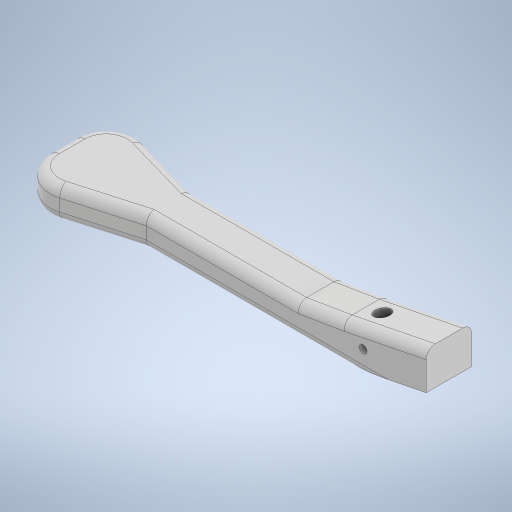
# Autodesk Inventor part: ручка печать
Saved by Autodesk Inventor 2023 (Build 270158000, 158)
## iProperties
Created: 2022-04-24
Part Number: ручка печать
Material: Типовые
Document SubType Name: Modeling
Designer: avkap
Density: 1 g/cm^3
Appearance: По умолчанию
Author: avkap
Autodesk Inventor part; units mm, degrees
ref_plane "YZ Plane" through (0, 0, 0) normal (1, 0, 0) x (0, 1, 0)
ref_plane "XZ Plane" through (0, 0, 0) normal (0, 1, 0) x (-1, 0, 0)
ref_plane "XY Plane" through (0, 0, 0) normal (0, 0, 1) x (1, 0, 0)
sketch "Эскиз1" plane through (0, 0, 0) normal (0, 1, 0) x (-1, 0, 0)
  line L0 (-70, 0) -> (-200, 0)
  line L1 (-200, 0) -> (-200, -30)
  line L2 (-200, -30) -> (0, -30)
  line L3 (0, -30) -> (0, 0)
  line L4 (0, 0) -> (0, 20)
  line L5 (0, -30) -> (0, -50)
  line L6 (0, 0) -> (-70, 0)
  line L7 (-70, 0) -> (0, 20)
  line L8 (-70, 0) -> (-70, -30)
  line L9 (0, -50) -> (-70, -30)
  dimension "d0" = 200
  dimension "d1" = 30
  dimension "d2" = 20
  dimension "d3" = 20
  dimension "d4" = 70
  constraints: 20 end point, 2 parallel, 2 perpendicular, 2 point on line, 1 horizontal, 1 vertical
  measures "d0" distance of L2.end L1.end
  measures "d1" distance of L2.end L3.end
  measures "d2" distance of L3.end L4.end
  measures "d3" distance of L2.end L5.end
  measures "d4" distance of L0.start L3.end
extrude "Выдавливание1" add sketch "Эскиз1" along normal blind 20
fillet "Сопряжение1" radius 20 2 edges at (0, 10, 20) (0, 10, -50)
ref_plane "РабПлоскость1" through (70.7003, 5, 0) normal (0, 0, 1) x (1, 0, 0)
sketch "Эскиз2" plane through (70.7003, 5, 0) normal (0, 0, 1) x (1, 0, 0)
  arc A0 (124.2997, -5) -> (129.2997, 0) centre (124.2997, 0) ccw projected
  line L0 (124.2997, 15) -> (0, 15) projected
  line L1 (124.2997, -5) -> (124.2997, 15)
  line L2 (124.2997, -5) -> (0, -5) projected
  line L3 (124.2997, -5) -> (154.2997, -5)
  line L4 (154.2997, -5) -> (154.2997, 15)
  line L5 (154.2997, 15) -> (124.2997, 15)
  line L6 (129.2997, -5) -> (129.2997, 15)
  line L7 (129.2997, 15) -> (129.2997, 20)
  line L8 (129.2997, 20) -> (154.2997, 20)
  line L9 (154.2997, 20) -> (154.2997, 15)
  line L10 (129.2997, -5) -> (154.2997, 0)
  line L11 (154.2997, 20) -> (129.2997, 15)
  line L12 (154.2997, 0) -> (184.2997, 0)
  line L13 (184.2997, 0) -> (184.2997, 15)
  line L14 (184.2997, 15) -> (154.2997, 15)
  line L15 (154.2997, 15) -> (154.2997, 0)
  line L16 (154.2997, 0) -> (184.2997, 6)
  line L17 (154.2997, 20) -> (184.2997, 26)
  line L18 (184.2997, 26) -> (184.2997, 15)
  line L19 (124.2997, 15) -> (124.2997, 20)
  line L20 (124.2997, 20) -> (129.2997, 20)
  line L21 (184.2997, 26) -> (184.2997, 31)
  line L22 (124.2997, 15) -> (124.2997, 10) projected
  line L23 (184.2997, 31) -> (129.2997, 20)
  line L24 (129.2997, 15) -> (99.2997, 15)
  line L25 (99.2997, 15) -> (129.2997, 20)
  point P0 (-70.7003, -5)
  dimension "d10" = 30
  dimension "d11" = 5
  dimension "d19" = 30
  dimension "d24" = 5
  dimension "d25" = 30
  constraints: 46 end point, 9 point on line, 8 perpendicular, 4 parallel, 2 vertical, 1 collinear, 1 horizontal
  measures "d10" distance of L1.start L3.end
  measures "d11" distance of L6.end L7.end
  measures "d19" distance of L14.end L13.end
  measures "d24" distance of L17.end L21.end
  measures "d25" distance of L6.end L24.end
extrude "Выдавливание2" add sketch "Эскиз2" against normal blind 30 contours L1 L5 L6 A0 | A0 L6 L3 | L6 L5 L4 L10 | L11 L9 L5 | L5 L19 L25 L7 | L7 L8 L11 | L0 L25 L19 | L4 L14 L13 L16 | L9 L17 L18 L14 | L23 L21 L17 L8
sketch "Эскиз4" plane through (255, 11, -30) normal (0.1961161, -0.9805807, 0) x (0.9805807, 0.1961161, 0)
  point P0 (-252.2053, 30)
ref_plane "РабПлоскость2" through (255, 11, -30) normal (0.1961161, -0.9805807, 0) x (0.9805807, 0.1961161, 0)
sketch "Эскиз5" plane through (255, 11, -30) normal (0.1961161, -0.9805807, 0) x (0.9805807, 0.1961161, 0)
  line L0 (-56.0892, 25) -> (-56.0892, 5) projected
  line L1 (-56.0892, 15) -> (0, 15)
  line L2 (0, 30) -> (0, 0) projected
  line L3 (0, 15) -> (-10, 15)
  circle A0 centre (-10, 15) radius 6
  point P0 (-252.2053, 30)
  dimension "d20" = 10
  dimension "d21" = 12
  constraints: 4 end point, 2 midpoint, 1 centre point, 1 coincident, 1 point on line
  measures "d20" distance of L1.end L3.end
  measures "d21" diameter of A0
sketch "Эскиз6" plane through (200, 0, -30) normal (0.1961161, -0.9805807, 0) x (0.9805807, 0.1961161, 0)
  circle A0 centre (46.0892, 15) radius 6 projected
  line L0 (46.0892, 15) -> (16.0892, 15)
  circle A1 centre (16.0892, 15) radius 5
  point P0 (-196.1161, 30)
  dimension "d26" = 30
  dimension "d27" = 10
  constraints: 2 end point, 1 centre point, 1 coincident, 1 horizontal
  measures "d26" distance of L0.start L0.end
  measures "d27" diameter of A1
extrude "Выдавливание5" cut sketch "Эскиз6" against normal blind 61.75 contours A1
hole "Отверстие1" at (245.1942, 9.0388, -15) direction (-0.1961161, 0.9805807, 0) diameter 12 depth 17 tip angle 118
fillet "Сопряжение5" radius 6 19 edges at (185, 22.5, -30) (227.5, 30.5, -30) (227.5, 30.5, 0) (185, 22.5, 0) (120, 20, -30) (120, 20, 0) (7.9561, 20, -39.4524) (0, 20, -15) (7.9561, 20, 9.4524) (47.7472, 20, 6.3579) (47.7472, 20, -36.3579) (7.9561, 0, -39.4524) (0, 0, -15) (7.9561, 0, 9.4524) (47.7472, 0, 6.3579) (47.7472, 0, -36.3579) (135, 0, -30) (135, 0, 0) (200, 0, -15)
sketch "Эскиз7" plane through (255, 11, 0) normal (0, 0, 1) x (1, 0, 0)
  line L0 (-48.9338, 15.2132) -> (-39.128, 17.1744) projected
  line L1 (-34.3203, -6.8641) -> (-44.1261, -8.8252) projected
  line L2 (-44.0309, 16.1938) -> (-39.2232, -7.8446)
  circle A0 centre (-41.6271, 4.1746) radius 2.5
  point P0 (-255, -11)
  dimension "d38" = 5
  constraints: 3 midpoint, 2 end point, 1 centre point
  measures "d38" diameter of A0
extrude "Выдавливание6" cut sketch "Эскиз7" against normal blind 40
sketch "Эскиз8" plane through (255, 11, 0) normal (0, 0, 1) x (1, 0, 0)
  circle A0 centre (-41.6271, 4.1746) radius 2.5 projected
  line L0 (-25, -5) -> (-54.4174, -10.8835) projected
  line L1 (0, 25) -> (-55, 14) projected
  line L2 (-53.9182, 8.0975) -> (-55, 14) projected
  line L3 (-55, 14) -> (0, 25)
  line L4 (-25, -5) -> (0, 0) projected
  line L5 (0, 0) -> (-54.4174, -10.8835)
  circle A1 centre (-41.6271, 4.1746) radius 2.5
  line L6 (-41.6271, 4.1746) -> (-44.0309, 16.1938)
  line L7 (-55, 14) -> (0, 25) projected
  line L8 (-41.6271, 4.1746) -> (-39.2232, -7.8446)
  point P0 (-255, -11)
  dimension "d41" = 12.2573
  dimension "d42" = 12.2573
  constraints: 8 end point, 3 perpendicular, 2 point on line, 1 centre point, 1 coincident, 1 collinear, 1 concentric
  measures "d41" distance of L6.start L6.end
  measures "d42" distance of L6.start L8.end
